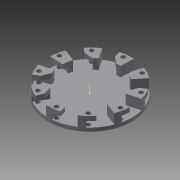
# Autodesk Inventor part: male bayonet connector 10
Saved by Autodesk Inventor 2015 (Build 190159000, 159)
## iProperties
Created: 2014-06-11
Part Number: male bayonet connector 10
Material: Generic
Document SubType Name: Modeling
Designer: ericd_000
Density: 1 g/cm^3
Appearance: Default
Author: ericd_000
Autodesk Inventor part; units mm, degrees
ref_plane "YZ Plane" through (0, 0, 0) normal (1, 0, 0) x (0, 1, 0)
ref_plane "XZ Plane" through (0, 0, 0) normal (0, 1, 0) x (-1, 0, 0)
ref_plane "XY Plane" through (0, 0, 0) normal (0, 0, 1) x (1, 0, 0)
sketch "Sketch19" plane through (0, 0, 0) normal (0, 0, 1) x (1, 0, 0)
  circle A0 centre (0, 0) radius 59
  dimension "d94" = 118
  constraints: 1 centre point, 1 coincident
  measures "d94" diameter of A0
extrude "Extrusion20" add sketch "Sketch19" along normal blind 5
sketch "Sketch21" plane through (0, 0, 5) normal (0, 0, 1) x (1, 0, 0)
  point P0 (0, 0)
sketch "Sketch23" plane through (0, 0, 5) normal (0, 0, 1) x (1, 0, 0)
  line L0 (0, 0) -> (30.298, 50.6264) construction
  circle A0 centre (0, 0) radius 59 construction
  line L1 (0, 0) -> (37.049, 45.917) construction
  circle A1 centre (0, 0) radius 59 construction
  line L2 (37.049, 45.917) -> (25.7528, 31.917)
  line L3 (25.7528, 31.917) -> (20.8552, 34.848)
  line L4 (20.8552, 34.848) -> (30.298, 50.6264)
  arc A2 (37.049, 45.917) -> (30.298, 50.6264) centre (0, 0) ccw
  dimension "d105" = 172
  dimension "d106" = 14
  constraints: 10 end point, 2 collinear, 2 point on circle, 1 centre point, 1 perpendicular, 5 other
  measures "d105" angle of L0 L1
  measures "d106" vertical distance of L1.end L2.end
extrude "Extrusion21" add sketch "Sketch23" along normal blind 14
sketch "Sketch26" plane through (20.8552, 34.848, 5) normal (-0.8580744, 0.5135254, 0) x (0, 0, 1)
  line L0 (14, 18.3881) -> (14, 0)
  line L1 (14, 18.3881) -> (8, 18.3881)
  line L2 (0, 18.3881) -> (14, 18.3881) projected
  line L3 (0, 0) -> (14, 0) projected
  line L4 (8, 0) -> (14, 0)
  line L5 (8, 18.3881) -> (8, 0)
  line L6 (-9, -40.6119) -> (19, -40.6119) projected
  point P0 (-5, -40.6119)
  dimension "d122" = 6
  dimension "d123" = 6
  constraints: 8 end point, 2 point on line, 1 collinear, 1 vertical
  measures "d122" distance of L0.start L1.end
  measures "d123" distance of L4.start L0.end
revolve "Revolution2" add sketch "Sketch26" angle 10 about axis through (0, 0, 5) along (0, 0, 1)
sketch "Sketch25" plane through (0, 0, 19) normal (0, 0, 1) x (1, 0, 0)
  circle A0 centre (26.0828, 47.2831) radius 3
  line L0 (26.0828, 47.2831) -> (0, 0) construction
  line L1 (14.4871, 37.9401) -> (21.0465, 55.1185) projected
  dimension "d112" = 6
  dimension "d116" = 54
  dimension "d125" = 7.5
  constraints: 2 end point, 1 centre point
  measures "d112" diameter of A0
  measures "d116" distance of L0.start L0.end
  measures "d125" distance from line of L0.start L1
extrude "Extrusion22" cut sketch "Sketch25" against normal through all
sketch "Sketch27" plane through (0, 0, 19) normal (0, 0, 1) x (1, 0, 0)
  line L0 (14.4871, 37.9401) -> (21.0465, 55.1185) projected
  line L1 (17.7668, 46.5293) -> (20.8552, 34.848)
  line L2 (20.8552, 34.848) -> (25.7528, 31.917) projected
  line L3 (14.4871, 37.9401) -> (17.7668, 46.5293)
  line L4 (20.8552, 34.848) -> (14.4871, 37.9401)
  point P0 (0, 0)
  constraints: 7 end point, 1 collinear, 1 midpoint
extrude "Extrusion23" cut sketch "Sketch27" against normal blind 10
pattern_circular "Circular Pattern2" count 10 over 360 about axis through (0, 0, 5) along (0, 0, 1) of "Extrusion21", "Revolution2", "Extrusion22", "Extrusion23"
sketch "Sketch28" plane through (0, 0, 19) normal (0, 0, 1) x (0.9785128, -0.2061861, 0)
  line L0 (-49.1928, -7.7914) -> (-40.1119, -6.3531)
  line L1 (-40.6057, 0.7088) -> (-49.1928, -7.7914)
  line L2 (-49.1928, -7.7914) -> (-40.6057, 0.7088) projected
  arc A0 (-40.6057, 0.7088) -> (-40.1119, -6.3531) centre (0, 0) ccw
  arc A1 (-58.2736, 9.2296) -> (-58.2736, -9.2296) centre (0, 0) ccw projected
  line L3 (-49.1928, -7.7914) -> (-58.2736, -9.2296) projected
  constraints: 4 end point, 2 collinear, 2 point on circle, 1 centre point, 1 concentric
extrude "Extrusion24" add sketch "Sketch28" against normal blind 6
body "Solid2"
